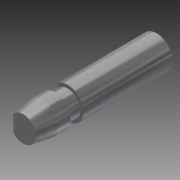
# Autodesk Inventor part: Lg Motor Shaft
Saved by Autodesk Inventor 2013 (Build 170138000, 138)
## iProperties
Created: 2014-08-02
Part Number: Lg Motor Shaft
Material: Stainless Steel
Document SubType Name: Modeling
Designer: Kyle
Density: 1 g/cm^3
Author: Kyle
Autodesk Inventor part; units mm, degrees
ref_plane "YZ Plane" through (0, 0, 0) normal (1, 0, 0) x (0, 1, 0)
ref_plane "XZ Plane" through (0, 0, 0) normal (0, 1, 0) x (-1, 0, 0)
sketch "Sketch1" plane through (0, 0, 0) normal (0, 0, 1) x (1, 0, 0)
  circle A0 centre (0, 0) radius 1.5875
  dimension "d0" = 3.175
  constraints: 1 centre point, 1 coincident
  measures "d0" diameter of A0
extrude "Extrusion1" add sketch "Sketch1" along normal blind 3.81
sketch "Sketch2" plane through (0, 0, 3.81) normal (0, 0, 1) x (1, 0, 0)
  circle A0 centre (0, 0) radius 1.5875 projected
  line L0 (-0.9525, 1.27) -> (-0.9525, -1.27)
  arc A1 (-0.9525, -1.27) -> (-0.9525, 1.27) centre (0, 0) ccw
  point P0 (1.5875, 0)
  point P1 (-0.9525, 0)
  dimension "d4" = 2.54
  constraints: 6 point on circle, 2 end point, 1 centre point, 1 coincident, 1 vertical
  measures "d4" distance of point (-0.953, 0) A0.start
extrude "Extrusion2" add sketch "Sketch2" along normal blind 5.08 contours A0 L0 picked at (0.1068, 0.3913)
sketch "Sketch3" plane through (0, 0, 8.89) normal (0, 0, 1) x (1, 0, 0)
  arc A0 (-0.9525, -1.27) -> (-0.9525, 1.27) centre (0, 0) ccw projected
  line L0 (-0.9525, 1.27) -> (-0.9525, -1.27) projected
  arc A1 (-0.9525, -0.84) -> (-0.9525, 0.84) centre (0, 0) ccw
  line L1 (-0.9525, 0.84) -> (-0.9525, -0.84)
  dimension "d8" = 2.54
  constraints: 2 end point, 2 point on circle, 2 point on line, 1 centre point, 1 coincident
  measures "d8" diameter of A1
extrude "Extrusion3" add sketch "Sketch3" along normal blind 1.27 contours L0 A1
sketch "Sketch4" plane through (0, 0, 10.16) normal (0, 0, 1) x (1, 0, 0)
  line L0 (-0.9525, 0.84) -> (-0.9525, -0.84) projected
  arc A0 (-0.9525, -0.84) -> (-0.9525, 0.84) centre (0, 0) ccw projected
  arc A1 (-0.9525, -1.27) -> (-0.9525, 1.27) centre (0, 0) ccw
  line L1 (-0.9525, 1.27) -> (-0.9525, -1.27)
  dimension "d12" = 3.175
  constraints: 2 end point, 2 point on circle, 1 centre point, 1 coincident, 1 collinear
  measures "d12" diameter of A1
extrude "Extrusion4" add sketch "Sketch4" along normal blind 1.27
ref_plane "Work Plane1" through (0, 0, 13.335) normal (0, 0, 1) x (1, 0, 0)
sketch "Sketch5" plane through (0, 0, 13.335) normal (0, 0, 1) x (1, 0, 0)
  arc A0 (-0.9525, -0.84) -> (-0.9525, 0.84) centre (0, 0) ccw
  line L0 (-0.9525, 0.84) -> (-0.9525, -0.84)
  point P0 (1.5875, 0)
  point P1 (-0.9525, 0)
  dimension "d17" = 2.54
  dimension "d19" = 1.5875
  dimension "d20" = 2.54
  constraints: 2 end point, 2 point on circle, 1 centre point, 1 coincident, 1 vertical
  measures "d17" diameter of A0
  measures "d19" distance of point (1.587, 0) point (0, 0)
  measures "d20" distance of point (1.587, 0) point (-0.953, 0)
sketch "Sketch6" plane through (0, 0, 11.43) normal (0, 0, 1) x (1, 0, 0)
  arc A0 (-0.9525, -1.27) -> (-0.9525, 1.27) centre (0, 0) ccw projected
  line L0 (-0.9525, 1.27) -> (-0.9525, -1.27) projected
loft "Loft1" add profiles "Sketch5" section 1 edges at (1.5875, 0, 11.43) (-0.9525, 0, 11.43)
body "Solid1"
